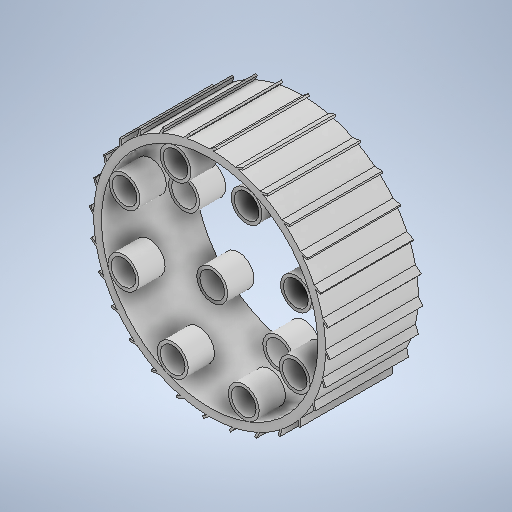
# Autodesk Inventor part: opona
Saved by Autodesk Inventor 2025.3 (Build 293356000, 356)
## iProperties
Created: 2026-03-13
Part Number: opona
Material: Generic
Document SubType Name: Modeling
Designer: ksawe
Density: 1 g/cm^3
Appearance: Default
Author: ksawe
Autodesk Inventor part; units mm, degrees
ref_plane "YZ Plane" through (0, 0, 0) normal (1, 0, 0) x (0, 1, 0)
ref_plane "XZ Plane" through (0, 0, 0) normal (0, 1, 0) x (-1, 0, 0)
ref_plane "XY Plane" through (0, 0, 0) normal (0, 0, 1) x (1, 0, 0)
sketch "Sketch1" plane through (0, 0, 0) normal (0, 0, 1) x (1, 0, 0)
  circle A0 centre (0, 0) radius 75
  circle A1 centre (0, 0) radius 70
  dimension "d0" = 150
  dimension "d1" = 140
  constraints: 2 centre point, 2 coincident
  measures "d0" diameter of A0
  measures "d1" diameter of A1
extrude "Extrusion1" add sketch "Sketch1" along normal mid plane 60
sketch "Sketch2" plane through (0, 0, 30) normal (0, 0, 1) x (1, 0, 0)
  circle A0 centre (0, 0) radius 50
  circle A1 centre (0, 0) radius 70 projected
  circle A2 centre (1, 60) radius 10
  circle A3 centre (1, 60) radius 8
  circle A4 centre (-22.0371, 55.8155) radius 8
  circle A5 centre (-22.0371, 55.8155) radius 10
  circle A6 centre (-41.7193, 43.1335) radius 8
  circle A7 centre (-41.7193, 43.1335) radius 10
  circle A8 centre (-55.0501, 23.8849) radius 8
  circle A9 centre (-55.0501, 23.8849) radius 10
  circle A10 centre (-60, 1) radius 8
  circle A11 centre (-60, 1) radius 10
  circle A12 centre (-55.8155, -22.0371) radius 8
  circle A13 centre (-55.8155, -22.0371) radius 10
  circle A14 centre (-43.1335, -41.7193) radius 8
  circle A15 centre (-43.1335, -41.7193) radius 10
  circle A16 centre (-23.8849, -55.0501) radius 8
  circle A17 centre (-23.8849, -55.0501) radius 10
  circle A18 centre (-1, -60) radius 8
  circle A19 centre (-1, -60) radius 10
  circle A20 centre (22.0371, -55.8155) radius 8
  circle A21 centre (22.0371, -55.8155) radius 10
  circle A22 centre (41.7193, -43.1335) radius 8
  circle A23 centre (41.7193, -43.1335) radius 10
  circle A24 centre (55.0501, -23.8849) radius 8
  circle A25 centre (55.0501, -23.8849) radius 10
  circle A26 centre (60, -1) radius 8
  circle A27 centre (60, -1) radius 10
  circle A28 centre (55.8155, 22.0371) radius 8
  circle A29 centre (55.8155, 22.0371) radius 10
  circle A30 centre (43.1335, 41.7193) radius 8
  circle A31 centre (43.1335, 41.7193) radius 10
  circle A32 centre (23.8849, 55.0501) radius 8
  circle A33 centre (23.8849, 55.0501) radius 10
  point P0 (0.7257, 69.9962)
  point P1 (1.6072, 69.9815)
  point P2 (-26.1159, 64.9458)
  point P3 (-25.2959, 65.2696)
  point P4 (-48.3479, 50.6209)
  point P5 (-48.9817, 50.008)
  point P6 (-64.0395, 28.2657)
  point P7 (-64.3904, 27.4569)
  point P8 (-69.9815, 1.6072)
  point P9 (-69.9962, 0.7257)
  point P10 (-65.2696, -25.2959)
  point P11 (-64.9458, -26.1159)
  point P12 (-27.4569, -64.3904)
  point P13 (-28.2657, -64.0395)
  point P14 (-50.008, -48.9817)
  point P15 (-50.6209, -48.3479)
  point P16 (25.2959, -65.2696)
  point P17 (26.1159, -64.9458)
  point P18 (64.0395, -28.2657)
  point P19 (64.3904, -27.4569)
  point P20 (64.9458, 26.1159)
  point P21 (65.2696, 25.2959)
  point P22 (27.4569, 64.3904)
  point P23 (28.2657, 64.0395)
  dimension "d4" = 100
  dimension "d10" = 2
  dimension "d13" = 360
  dimension "d52" = 60
  dimension "d53" = 22.8849
  dimension "d87" = 20
  constraints: 33 centre point, 3 coincident, 50 other
  measures "d4" diameter of A0
  measures "d10" radial gap between concentric circles of A2 A3
  measures "d52" vertical distance of point (0, 0) A2.centre
  measures "d53" horizontal distance of A32.centre A2.centre
  measures "d87" diameter of A2
extrude "Extrusion3" add sketch "Sketch2" against normal blind 17 contours A29 A1 | A1 A25 | A33 A1 | A1 A21 | A5 A1 | A1 A17 | A9 A1 | A1 A13 picked at (64.9724, 20.5927) picked at (64.2081, -22.445) picked at (33.0438, 53.6138) picked at (31.2747, -55.0225) picked at (-12.7981, 55.0282) picked at (-14.7262, -56.4871) picked at (-45.8933, 25.3296) picked at (-46.6617, -20.5804)
sketch "Sketch4" plane through (0, 0, -30) normal (0, 0, -1) x (-1, 0, 0)
  circle A0 centre (-0.4184, -0.251) radius 50
  circle A1 centre (-0.4184, -0.251) radius 70
  circle A2 centre (0.5816, 59.749) radius 10
  circle A3 centre (0.5816, 59.749) radius 8
  circle A4 centre (-22.4555, 55.5644) radius 8
  circle A5 centre (-22.4555, 55.5644) radius 10
  circle A6 centre (-42.1377, 42.8825) radius 8
  circle A7 centre (-42.1377, 42.8825) radius 10
  circle A8 centre (-55.4685, 23.6338) radius 8
  circle A9 centre (-55.4685, 23.6338) radius 10
  circle A10 centre (-60.4184, 0.749) radius 8
  circle A11 centre (-60.4184, 0.749) radius 10
  circle A12 centre (-56.2339, -22.2882) radius 8
  circle A13 centre (-56.2339, -22.2882) radius 10
  circle A14 centre (-43.5519, -41.9703) radius 8
  circle A15 centre (-43.5519, -41.9703) radius 10
  circle A16 centre (-24.3033, -55.3011) radius 8
  circle A17 centre (-24.3033, -55.3011) radius 10
  circle A18 centre (-1.4184, -60.251) radius 8
  circle A19 centre (-1.4184, -60.251) radius 10
  circle A20 centre (21.6187, -56.0665) radius 8
  circle A21 centre (21.6187, -56.0665) radius 10
  circle A22 centre (41.3009, -43.3846) radius 8
  circle A23 centre (41.3009, -43.3846) radius 10
  circle A24 centre (54.6317, -24.1359) radius 8
  circle A25 centre (54.6317, -24.1359) radius 10
  circle A26 centre (59.5816, -1.251) radius 8
  circle A27 centre (59.5816, -1.251) radius 10
  circle A28 centre (55.397, 21.7861) radius 8
  circle A29 centre (55.397, 21.7861) radius 10
  circle A30 centre (42.7151, 41.4683) radius 8
  circle A31 centre (42.7151, 41.4683) radius 10
  circle A32 centre (23.4665, 54.799) radius 8
  circle A33 centre (23.4665, 54.799) radius 10
  point P0 (0, 0)
  point P1 (-70.4, 1.3562)
  point P2 (-70.4147, 0.4747)
  point P3 (-51.0393, -48.599)
  point P4 (-50.4264, -49.2327)
  point P5 (-1.1441, -70.2473)
  point P6 (-2.0257, -70.2326)
  point P7 (48.5632, -50.259)
  point P8 (47.9295, -50.872)
  point P9 (49.5896, 48.7306)
  point P10 (50.2025, 48.0969)
  point P11 (0.3073, 69.7452)
  point P12 (1.1888, 69.7305)
  point P13 (-49.4001, 49.7569)
  point P14 (-48.7664, 50.3699)
  dimension "d92" = 100
  dimension "d93" = 2
  dimension "d94" = 360
  dimension "d95" = 60
  dimension "d96" = 22.8849
  dimension "d97" = 20
  constraints: 34 centre point, 3 coincident, 49 other
  measures "d92" diameter of A0
  measures "d93" radial gap between concentric circles of A2 A3
  measures "d95" vertical distance of point (-0.418, -0.251) A2.centre
  measures "d96" horizontal distance of A32.centre A2.centre
  measures "d97" diameter of A2
extrude "Extrusion4" add sketch "Sketch4" against normal blind 17 contours A27 A1 | A1 A27 | A31 A1 | A1 A23 | A2 A1 | A1 A19 | A7 A1 | A1 A15 | A11 A1 picked at (51.8684, 40.0098) picked at (50.4555, -41.931) picked at (9.7366, 58.2972) picked at (7.738, -58.8049) picked at (-32.9804, 41.4399) picked at (-34.3154, -41.1726) picked at (-51.1803, -0.0419)
sketch "Sketch5" plane through (0, 0, 30) normal (0, 0, 1) x (1, 0, 0)
  circle A0 centre (0, 0) radius 75 projected
  line L0 (0, 75) -> (4, 78)
  line L1 (4, 78) -> (4.75, 77)
  line L2 (4.75, 77) -> (2.0461, 74.9721)
  constraints: 6 end point, 2 point on circle, 1 perpendicular
extrude "Extrusion5" add sketch "Sketch5" against normal blind 60 contours A0 L0 L1 L2
pattern_circular "Circular Pattern1" count 28 over 360 about axis through (0, 0, 0) along (0, 0, 1) of "Extrusion5"
body "Solid1"
